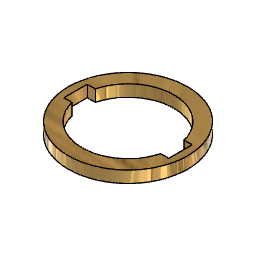
Centering ring with motor hook slots v8 (Autodesk Fusion 360 design; units mm, degrees)
Autodesk Fusion 360 part; units mm, degrees
sketch "Sketch1" plane through (0, 0, 0) normal (0, 0, 1) x (1, 0, 0)
  circle A0 centre (17.385, 5) radius 20.5
  line L0 (0, 8.75) -> (0, 8.6219)
  line L1 (-0.615, 1.25) -> (0, 1.3781) construction
  line L2 (0, 8.6219) -> (0, 8.75)
  line L3 (0, 1.25) -> (-0.615, 1.25)
  line L4 (-0.615, 1) -> (-0.615, 9)
  line L5 (35.385, 9) -> (35.385, 1)
  line L6 (-0.615, 9) -> (2.1514, 9)
  line L7 (32.6186, 9) -> (35.385, 9)
  line L8 (2.1514, 1) -> (-0.615, 1)
  arc A1 (2.1514, 1) -> (32.6186, 1) centre (17.385, 5) ccw
  arc A2 (32.6186, 9) -> (2.1514, 9) centre (17.385, 5) ccw
  line L9 (32.6186, 1) -> (35.385, 1)
  point P0 (17.385, 5)
  point P1 (17.385, 5)
  point P2 (17.385, 5)
  dimension "d4" = 41
  dimension "d11" = 36
  dimension "d12" = 8
  dimension "d13" = 31.5
  constraint vertical L0
  constraint coincident P2 L1
  constraint parallel L4 L5
  constraint coincident P2 P1
  constraint coincident L7.start A1
  constraint collinear L6 L7
  constraint concentric A1 A2
  constraint perpendicular L5 L9
  measures "d4" diameter of A0
  measures "d11" distance of L4.end L5.start
  measures "d12" distance of L4.start L4.end
  measures "d13" diameter of A1
extrude "Extrude1" add sketch "Sketch1" along normal blind 4
